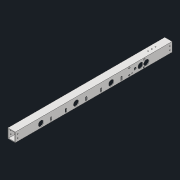
# Autodesk Inventor part: Left Frame
Saved by Autodesk Inventor 2022 (Build 260153000, 153)
## iProperties
Created: 2022-09-06
Part Number: Left Frame
Material: Generic
Document SubType Name: Modeling
Designer: robpl
Density: 1 g/cm^3
Appearance: Default
Author: robpl
Autodesk Inventor part; units mm, degrees
ref_plane "YZ Plane" through (0, 0, 0) normal (1, 0, 0) x (0, 1, 0)
ref_plane "XZ Plane" through (0, 0, 0) normal (0, 1, 0) x (-1, 0, 0)
sketch "Sketch1" plane through (0, 0, 0) normal (0, 0, 1) x (1, 0, 0)
  line L0 (0, 0) -> (40, 0)
  line L1 (40, 0) -> (40, 50)
  line L2 (40, 50) -> (0, 50)
  line L3 (0, 50) -> (0, 0)
  line L4 (37, 47) -> (37, 3)
  line L5 (37, 3) -> (3, 3)
  line L6 (3, 3) -> (3, 47)
  line L7 (3, 47) -> (37, 47)
  dimension "d0" = 40
  dimension "d1" = 50
  dimension "d2" = 3
  constraints: 16 end point, 4 parallel, 2 perpendicular, 1 horizontal, 3 other
  measures "d0" distance of L2.end L1.end
  measures "d1" distance of L1.end L0.end
  measures "d2" distance between parallel lines of L1 L4
extrude "Extrusion1" add sketch "Sketch1" along normal blind 850
sketch "Sketch2" plane through (40, 0, 0) normal (1, 0, 0) x (0, 0, -1)
  line L0 (0, 0) -> (0, 50) projected
  line L1 (0, 50) -> (-850, 50) projected
  line L2 (-850, 0) -> (-850, 50) projected
  line L3 (0, 0) -> (-850, 0) projected
  point P0 (-710.75, 21)
  point P1 (-520.25, 21)
  point P2 (-329.75, 21)
  point P3 (-139.25, 21)
  dimension "d5" = 190.5
  dimension "d6" = 190.5
  dimension "d7" = 190.5
  dimension "d8" = 850
  dimension "d9" = 139.25
  dimension "d10" = 21
  constraints: 3 horizontal alignment
  measures "d5" distance of point (-329.75, 21) point (-139.25, 21)
  measures "d6" distance of point (-520.25, 21) point (-329.75, 21)
  measures "d7" distance of point (-710.75, 21) point (-520.25, 21)
  measures "d8" distance of L0.end L1.end
  measures "d9" distance from line of point (-139.25, 21) L0
  measures "d10" distance from line of L3 point (-139.25, 21)
hole "Hole1" at (40, 21, 710.75) at (40, 21, 520.25) at (40, 21, 329.75) at (40, 21, 139.25) direction (-1, 0, 0) diameter 28.575 end through all
sketch "Sketch3" plane through (0, 0, 0) normal (0, -1, 0) x (1, 0, 0)
  line L0 (37, 0) -> (37, 850) projected
  line L1 (3, 0) -> (3, 850) projected
  line L2 (37, 755) -> (3, 755)
  line L3 (3, 755) -> (3, 95)
  line L4 (3, 95) -> (37, 95)
  line L5 (37, 95) -> (37, 755)
  line L6 (40, 725.0375) -> (40, 696.4625) projected
  line L7 (40, 0) -> (40, 850) projected
  line L8 (0, 850) -> (40, 850) projected
  line L9 (0, 0) -> (40, 0) projected
  point P0 (40, 710.75)
  point P1 (37, 95)
  point P2 (3, 755)
  dimension "d18" = 28.575
  dimension "d19" = 14.2875
  dimension "d22" = 95
  dimension "d23" = 95
  constraints: 8 end point, 3 point on line, 2 parallel, 1 horizontal, 1 perpendicular
  measures "d18" distance of L6.start L6.end
  measures "d19" distance of L6.start point (40, 710.75)
  measures "d22" distance between parallel lines of L8 L2
  measures "d23" distance between parallel lines of L9 L4
extrude "Extrusion2" cut sketch "Sketch3" against normal blind 3 contours L4 L1 L2 L0
sketch "Sketch4" plane through (40, 0, 0) normal (1, 0, 0) x (0, 0, -1)
  line L0 (-842.1969, 39.5285) -> (-10.8553, 39.5285)
  line L1 (-10.8553, 39.5285) -> (-10.8553, 6.7172)
  line L2 (-10.8553, 6.7172) -> (-842.1969, 6.7172)
  line L3 (-842.1969, 6.7172) -> (-842.1969, 39.5285)
  point P0 (0, 0)
  constraints: 8 end point, 2 parallel, 1 horizontal, 1 perpendicular
extrude "Extrusion3" [suppressed]
sketch "Sketch5" plane through (0, 0, 0) normal (-1, 0, 0) x (0, 0, 1)
  line L0 (0, 50) -> (0, 0) projected
  line L1 (0, 0) -> (850, 0) projected
  circle A0 centre (710.75, 21) radius 14.2875 projected
  circle A1 centre (139.25, 21) radius 14.2875 projected
  circle A2 centre (329.75, 21) radius 14.2875 projected
  circle A3 centre (520.25, 21) radius 14.2875 projected
  line L2 (0, 0) -> (0, 50) projected
  line L3 (0, 50) -> (850, 50) projected
  line L4 (850, 0) -> (850, 50) projected
  line L5 (0, 0) -> (850, 0) projected
  line L6 (139.25, 21) -> (107.5, 22.8)
  dimension "d37" = 31.801
  dimension "d39" = 107.5
  dimension "d41" = 22.8
  constraints: 2 end point, 1 coincident
  measures "d37" distance of L6.start L6.end
  measures "d39" distance from line of L0 L6.end
  measures "d41" distance from line of L1 L6.end
hole "Hole2" at (0, 22.8, 107.5) direction (1, 0, 0) diameter 28.575 end through all
sketch "Sketch6" plane through (40, 0, 0) normal (1, 0, 0) x (0, 0, -1)
  circle A0 centre (-107.5, 22.8) radius 14.2875 projected
  circle A1 centre (-329.75, 21) radius 14.2875 projected
  circle A2 centre (-710.75, 21) radius 14.2875 projected
  circle A3 centre (-520.25, 21) radius 14.2875 projected
  circle A4 centre (-139.25, 21) radius 14.2875 projected
  line L0 (0, 3) -> (0, 47) projected
  line L1 (0, 47) -> (-850, 47) projected
  line L2 (-850, 3) -> (-850, 47) projected
  line L3 (-755, 3) -> (-850, 3) projected
  line L4 (-755, 0) -> (-755, 3) projected
  line L5 (-95, 0) -> (-755, 0) projected
  line L6 (-95, 0) -> (-95, 3) projected
  line L7 (0, 3) -> (-95, 3) projected
  point P0 (0, 0)
  point P1 (-78.24, 22.8)
  dimension "d42" = 29.26
  constraints: 1 horizontal alignment
  measures "d42" distance of A0.centre point (-78.24, 22.8)
hole "Hole3" at (40, 22.8, 78.24) direction (-1, 0, 0) diameter 13 end through all
sketch "Sketch9" plane through (40, 0, 0) normal (1, 0, 0) x (0, 0, -1)
  point P0 (0, 0)
  point P1 (-127.5, 42)
  point P2 (-46.5, 42)
  point P3 (-46.5, 8)
  point P4 (-125.5, 5)
  dimension "d78" = 5
  dimension "d79" = 8
  dimension "d80" = 42
  dimension "d81" = 46.5
  dimension "d82" = 81
  dimension "d83" = 79
  constraints: 1 horizontal alignment, 1 vertical alignment
  measures "d78" vertical distance of point (0, 0) point (-125.5, 5)
  measures "d79" vertical distance of point (0, 0) point (-46.5, 8)
  measures "d80" vertical distance of point (0, 0) point (-46.5, 42)
  measures "d81" horizontal distance of point (0, 0) point (-46.5, 8)
  measures "d82" horizontal distance of point (-127.5, 42) point (-46.5, 8)
  measures "d83" horizontal distance of point (-125.5, 5) point (-46.5, 8)
hole "Hole7" at (40, 42, 127.5) at (40, 42, 46.5) at (40, 8, 46.5) at (40, 5, 125.5) direction (-1, 0, 0) diameter 9 depth 8 tip angle 118
sketch "Sketch10" plane through (3, 3, 0) normal (1, 0, 0) x (0, 0, -1)
  circle A0 centre (-125.5, 2) radius 4.5 projected
  circle A1 centre (-127.5, 39) radius 4.5 projected
  circle A2 centre (-46.5, 39) radius 4.5 projected
  circle A3 centre (-46.5, 5) radius 4.5 projected
  point P0 (0, -3)
  constraints: 4 coincident
hole "Hole8" at (3, 5, 125.5) at (3, 42, 127.5) at (3, 42, 46.5) at (3, 8, 46.5) direction (-1, 0, 0) diameter 4 end through all countersink diameter 9 countersink angle 90
sketch "Sketch11" plane through (0, 0, 0) normal (0, -1, 0) x (1, 0, 0)
  point P0 (0, 0)
  point P1 (20, 51.5)
  point P2 (20, 86.5)
  dimension "d98" = 35
  dimension "d99" = 51.5
  dimension "d100" = 20
  constraints: 1 vertical alignment
  measures "d98" distance of point (20, 51.5) point (20, 86.5)
  measures "d99" vertical distance of point (0, 0) point (20, 51.5)
  measures "d100" horizontal distance of point (0, 0) point (20, 51.5)
hole "Hole9" at (20, 0, 51.5) at (20, 0, 86.5) direction (0, 1, 0) diameter 6 depth 8 tip angle 118
sketch "Sketch12" plane through (40, 0, 0) normal (1, 0, 0) x (0, 0, -1)
  point P0 (0, 0)
  point P1 (-12.5, 15)
  point P2 (-12.5, 35)
  point P3 (-837.5, 35)
  point P4 (-837.5, 15)
  dimension "d108" = 12.5
  dimension "d109" = 35
  dimension "d110" = 15
  dimension "d111" = 837.5
  constraints: 2 horizontal alignment, 2 vertical alignment
  measures "d108" horizontal distance of point (-12.5, 35) point (0, 0)
  measures "d109" vertical distance of point (0, 0) point (-12.5, 35)
  measures "d110" vertical distance of point (0, 0) point (-12.5, 15)
  measures "d111" horizontal distance of point (0, 0) point (-837.5, 15)
hole "Hole10" at (40, 15, 12.5) at (40, 35, 12.5) at (40, 35, 837.5) at (40, 15, 837.5) direction (-1, 0, 0) diameter 6 end through all
sketch "Sketch13" plane through (0, 0, 0) normal (-1, 0, 0) x (0, 0, 1)
  line L0 (0, 0) -> (850, 0) projected
  point P0 (245, 12.5)
  point P1 (425, 12.5)
  point P2 (605, 12.5)
  dimension "d119" = 180
  dimension "d120" = 180
  dimension "d121" = 12.5
  dimension "d122" = 425
  constraints: 2 horizontal alignment
  measures "d119" distance of point (425, 12.5) point (605, 12.5)
  measures "d120" distance of point (245, 12.5) point (425, 12.5)
  measures "d121" distance from line of L0 point (245, 12.5)
  measures "d122" horizontal distance of L0.start point (425, 12.5)
hole "Hole11" at (0, 12.5, 245) at (0, 12.5, 425) at (0, 12.5, 605) direction (1, 0, 0) diameter 5 depth 8 tip angle 118
sketch "Sketch14" plane through (40, 0, 0) normal (1, 0, 0) x (0, 0, -1)
  line L0 (-655.75, 21) -> (-655.75, 8) construction
  line L1 (-659.75, 21) -> (-659.75, 8)
  line L2 (-651.75, 8) -> (-651.75, 21)
  arc A0 (-651.75, 21) -> (-659.75, 21) centre (-655.75, 21) ccw
  arc A1 (-659.75, 8) -> (-651.75, 8) centre (-655.75, 8) ccw
  line L3 (0, 0) -> (-850, 0) projected
  circle A2 centre (-837.5, 35) radius 3 projected
  circle A3 centre (-12.5, 15) radius 3 projected
  circle A4 centre (-12.5, 35) radius 3 projected
  circle A5 centre (-837.5, 15) radius 3 projected
  circle A6 centre (-46.5, 8) radius 4.5 projected
  circle A7 centre (-127.5, 42) radius 4.5 projected
  circle A8 centre (-46.5, 42) radius 4.5 projected
  circle A9 centre (-125.5, 5) radius 4.5 projected
  circle A10 centre (-78.24, 22.8) radius 6.5 projected
  circle A11 centre (-107.5, 22.8) radius 14.2875 projected
  circle A12 centre (-329.75, 21) radius 14.2875 projected
  circle A13 centre (-710.75, 21) radius 14.2875 projected
  circle A14 centre (-520.25, 21) radius 14.2875 projected
  circle A15 centre (-139.25, 21) radius 14.2875 projected
  line L4 (0, 0) -> (0, 50) projected
  line L5 (0, 50) -> (-850, 50) projected
  line L6 (-850, 0) -> (-850, 50) projected
  line L7 (0, 0) -> (-850, 0) projected
  line L8 (-575.25, 21) -> (-575.25, 8) construction
  line L9 (-571.25, 21) -> (-571.25, 8)
  line L10 (-579.25, 8) -> (-579.25, 21)
  arc A16 (-571.25, 21) -> (-579.25, 21) centre (-575.25, 21) ccw
  arc A17 (-579.25, 8) -> (-571.25, 8) centre (-575.25, 8) ccw
  line L11 (-465.25, 8) -> (-465.25, 21) construction
  line L12 (0, 47) -> (-850, 47) projected
  line L13 (-461.25, 8) -> (-461.25, 21)
  line L14 (-469.25, 21) -> (-469.25, 8)
  arc A18 (-469.25, 8) -> (-461.25, 8) centre (-465.25, 8) ccw
  arc A19 (-461.25, 21) -> (-469.25, 21) centre (-465.25, 21) ccw
  line L15 (-384.75, 8) -> (-384.75, 21) construction
  line L16 (-388.75, 8) -> (-388.75, 21)
  line L17 (-380.75, 21) -> (-380.75, 8)
  arc A20 (-388.75, 8) -> (-380.75, 8) centre (-384.75, 8) ccw
  arc A21 (-380.75, 21) -> (-388.75, 21) centre (-384.75, 21) ccw
  line L18 (-274.75, 21) -> (-274.75, 8) construction
  line L19 (-270.75, 21) -> (-270.75, 8)
  line L20 (-278.75, 8) -> (-278.75, 21)
  arc A22 (-270.75, 21) -> (-278.75, 21) centre (-274.75, 21) ccw
  arc A23 (-278.75, 8) -> (-270.75, 8) centre (-274.75, 8) ccw
  line L21 (-194.25, 21) -> (-194.25, 8) construction
  line L22 (-190.25, 21) -> (-190.25, 8)
  line L23 (-198.25, 8) -> (-198.25, 21)
  arc A24 (-190.25, 21) -> (-198.25, 21) centre (-194.25, 21) ccw
  arc A25 (-198.25, 8) -> (-190.25, 8) centre (-194.25, 8) ccw
  point P0 (-655.75, 14.5)
  point P1 (-575.25, 14.5)
  point P2 (-465.25, 14.5)
  point P3 (-384.75, 14.5)
  point P4 (-274.75, 14.5)
  point P5 (-194.25, 14.5)
  dimension "d130" = 8
  dimension "d131" = 8
  dimension "d132" = 21
  dimension "d133" = 55
  dimension "d134" = 55
  dimension "d135" = 55
  dimension "d136" = 55
  dimension "d137" = 55
  dimension "d138" = 55
  constraints: 48 end point, 24 point on circle, 24 tangent, 14 parallel, 12 centre point, 6 midpoint, 5 equal radius, 5 horizontal alignment, 2 vertical, 1 perpendicular
  measures "d130" diameter of A1
  measures "d131" distance from line of L3 L0.end
  measures "d132" distance from line of L3 L0.start
  measures "d133" distance from line of L0 A13.centre
  measures "d134" horizontal distance of A14.centre point (-575.25, 14.5)
  measures "d135" distance from line of L11 A14.centre
  measures "d136" horizontal distance of A12.centre L15.start
  measures "d137" horizontal distance of A12.centre point (-274.75, 14.5)
  measures "d138" horizontal distance of A15.centre point (-194.25, 14.5)
extrude "Extrusion4" cut sketch "Sketch14" against normal through all contours A0 L2 A1 L1 | L9 A17 L10 A16 | A18 L14 A19 L13 | L16 A21 L17 A20 | L19 A23 L20 A22
ref_plane "Work Plane1" through (0, 0, 139.25) normal (0, 0, -1) x (-1, 0, 0)
mirror "Two Motors" about plane through (0, 0, 139.25) normal (0, 0, -1) of "Hole2", "Hole3", "Hole7", "Hole8"
sketch "Sketch16" plane through (40, 0, 0) normal (1, 0, 0) x (0, 0, -1)
  point P0 (0, 0)
  point P1 (-216.5, 10)
  dimension "d144" = 216.5
  dimension "d145" = 10
  measures "d144" horizontal distance of point (0, 0) point (-216.5, 10)
  measures "d145" vertical distance of point (0, 0) point (-216.5, 10)
hole "Two Motors b" at (40, 10, 216.5) direction (-1, 0, 0) diameter 6 end through all
sketch "Sketch18" plane through (40, 0, 0) normal (1, 0, 0) x (0, 0, -1)
  circle A0 centre (-216.5, 10) radius 3 projected
  circle A1 centre (-153, 5) radius 4.5 projected
  circle A2 centre (-232, 42) radius 4.5 projected
  circle A3 centre (-151, 42) radius 4.5 projected
  circle A4 centre (-232, 8) radius 4.5 projected
  circle A5 centre (-171, 22.8) radius 14.2875 projected
  circle A6 centre (-200.26, 22.8) radius 6.5 projected
  line L0 (-469.25, 8) -> (-469.25, 21) projected
  arc A7 (-461.25, 21) -> (-469.25, 21) centre (-465.25, 21) ccw projected
  line L1 (-461.25, 21) -> (-461.25, 8) projected
  arc A8 (-469.25, 8) -> (-461.25, 8) centre (-465.25, 8) ccw projected
  arc A9 (-388.75, 8) -> (-380.75, 8) centre (-384.75, 8) ccw projected
  line L2 (-388.75, 8) -> (-388.75, 21) projected
  arc A10 (-380.75, 21) -> (-388.75, 21) centre (-384.75, 21) ccw projected
  line L3 (-380.75, 21) -> (-380.75, 8) projected
  arc A11 (-571.25, 21) -> (-579.25, 21) centre (-575.25, 21) ccw projected
  line L4 (-571.25, 21) -> (-571.25, 8) projected
  arc A12 (-579.25, 8) -> (-571.25, 8) centre (-575.25, 8) ccw projected
  line L5 (-579.25, 8) -> (-579.25, 21) projected
  arc A13 (-270.75, 21) -> (-278.75, 21) centre (-274.75, 21) ccw projected
  line L6 (-270.75, 21) -> (-270.75, 8) projected
  arc A14 (-278.75, 8) -> (-270.75, 8) centre (-274.75, 8) ccw projected
  line L7 (-278.75, 8) -> (-278.75, 21) projected
  line L8 (-651.75, 21) -> (-651.75, 8) projected
  arc A15 (-659.75, 8) -> (-651.75, 8) centre (-655.75, 8) ccw projected
  line L9 (-659.75, 8) -> (-659.75, 21) projected
  arc A16 (-651.75, 21) -> (-659.75, 21) centre (-655.75, 21) ccw projected
  circle A17 centre (-837.5, 35) radius 3 projected
  circle A18 centre (-12.5, 15) radius 3 projected
  circle A19 centre (-12.5, 35) radius 3 projected
  circle A20 centre (-837.5, 15) radius 3 projected
  circle A21 centre (-46.5, 8) radius 4.5 projected
  circle A22 centre (-127.5, 42) radius 4.5 projected
  circle A23 centre (-46.5, 42) radius 4.5 projected
  circle A24 centre (-125.5, 5) radius 4.5 projected
  circle A25 centre (-78.24, 22.8) radius 6.5 projected
  circle A26 centre (-107.5, 22.8) radius 14.2875 projected
  circle A27 centre (-329.75, 21) radius 14.2875 projected
  circle A28 centre (-710.75, 21) radius 14.2875 projected
  circle A29 centre (-520.25, 21) radius 14.2875 projected
  circle A30 centre (-139.25, 21) radius 14.2875 projected
  line L10 (0, 0) -> (0, 50) projected
  line L11 (0, 50) -> (-850, 50) projected
  line L12 (-850, 0) -> (-850, 50) projected
  line L13 (0, 0) -> (-850, 0) projected
extrude "Extrusion6" add sketch "Sketch18" against normal blind 3 contours A21 | A22 | A23 | A24 | A25 | A26
sketch "Sketch19" plane through (3, 3, 0) normal (1, 0, 0) x (0, 0, -1)
  circle A0 centre (-216.5, 7) radius 3 projected
  circle A1 centre (-153, 2) radius 4.5 projected
  circle A2 centre (-151, 39) radius 4.5 projected
  circle A3 centre (-232, 5) radius 4.5 projected
  circle A4 centre (-232, 39) radius 4.5 projected
  circle A5 centre (-171, 19.8) radius 14.2875 projected
  circle A6 centre (-200.26, 19.8) radius 6.5 projected
  line L0 (-469.25, 5) -> (-469.25, 18) projected
  arc A7 (-461.25, 18) -> (-469.25, 18) centre (-465.25, 18) ccw projected
  line L1 (-461.25, 18) -> (-461.25, 5) projected
  arc A8 (-469.25, 5) -> (-461.25, 5) centre (-465.25, 5) ccw projected
  arc A9 (-388.75, 5) -> (-380.75, 5) centre (-384.75, 5) ccw projected
  line L2 (-388.75, 5) -> (-388.75, 18) projected
  arc A10 (-380.75, 18) -> (-388.75, 18) centre (-384.75, 18) ccw projected
  line L3 (-380.75, 18) -> (-380.75, 5) projected
  arc A11 (-571.25, 18) -> (-579.25, 18) centre (-575.25, 18) ccw projected
  line L4 (-571.25, 18) -> (-571.25, 5) projected
  arc A12 (-579.25, 5) -> (-571.25, 5) centre (-575.25, 5) ccw projected
  line L5 (-579.25, 5) -> (-579.25, 18) projected
  arc A13 (-270.75, 18) -> (-278.75, 18) centre (-274.75, 18) ccw projected
  line L6 (-270.75, 18) -> (-270.75, 5) projected
  arc A14 (-278.75, 5) -> (-270.75, 5) centre (-274.75, 5) ccw projected
  line L7 (-278.75, 5) -> (-278.75, 18) projected
  line L8 (-651.75, 18) -> (-651.75, 5) projected
  arc A15 (-659.75, 5) -> (-651.75, 5) centre (-655.75, 5) ccw projected
  line L9 (-659.75, 5) -> (-659.75, 18) projected
  arc A16 (-651.75, 18) -> (-659.75, 18) centre (-655.75, 18) ccw projected
  circle A17 centre (-425, 9.5) radius 2.5 projected
  circle A18 centre (-245, 9.5) radius 2.5 projected
  circle A19 centre (-605, 9.5) radius 2.5 projected
  circle A20 centre (-837.5, 32) radius 3 projected
  circle A21 centre (-12.5, 12) radius 3 projected
  circle A22 centre (-12.5, 32) radius 3 projected
  circle A23 centre (-837.5, 12) radius 3 projected
  circle A24 centre (-46.5, 39) radius 4.5 projected
  circle A25 centre (-125.5, 2) radius 4.5 projected
  circle A26 centre (-127.5, 39) radius 4.5 projected
  circle A27 centre (-46.5, 5) radius 4.5 projected
  circle A28 centre (-78.24, 19.8) radius 6.5 projected
  circle A29 centre (-107.5, 19.8) radius 14.2875 projected
  circle A30 centre (-329.75, 18) radius 14.2875 projected
  circle A31 centre (-710.75, 18) radius 14.2875 projected
  circle A32 centre (-520.25, 18) radius 14.2875 projected
  circle A33 centre (-139.25, 18) radius 14.2875 projected
  line L10 (0, 0) -> (0, 44) projected
  line L11 (0, 44) -> (-850, 44) projected
  line L12 (-850, 0) -> (-850, 44) projected
  line L13 (-755, 0) -> (-850, 0) projected
  line L14 (-755, -3) -> (-755, 0) projected
  line L15 (-95, -3) -> (-755, -3) projected
  line L16 (-95, -3) -> (-95, 0) projected
  line L17 (0, 0) -> (-95, 0) projected
  point P0 (0, -3)
extrude "Extrusion7" add sketch "Sketch19" against normal blind 3 contours A24 | A25 | A26 | A27 | A28 | A29
sketch "Sketch20" plane through (0, 50, 0) normal (0, 1, 0) x (1, 0, 0)
  point P0 (0, 0)
  point P1 (20, -110)
  point P2 (20, -90)
  point P3 (20, -70)
  dimension "d168" = 70
  dimension "d169" = 20
  dimension "d170" = 20
  dimension "d171" = 20
  constraints: 2 vertical alignment
  measures "d168" vertical distance of point (0, 0) point (20, -70)
  measures "d169" distance of point (20, -90) point (20, -70)
  measures "d170" distance of point (20, -110) point (20, -90)
  measures "d171" horizontal distance of point (0, 0) point (20, -70)
hole "Hole14" at (20, 50, 110) at (20, 50, 90) at (20, 50, 70) direction (0, -1, 0) diameter 5 depth 8 tip angle 118
equation "\"d6\" = d5"
equation "\"d7\" = d5"
equation "\"d9\" = -1.5 * d5 + 0.5 * d8"
equation "\"d19\" = 0.5 * d18"
equation "\"d120\" = d119"
equation "\"d134\" = d133"
equation "\"d135\" = d133"
equation "\"d136\" = d133"
equation "\"d137\" = d133"
equation "\"d138\" = d133"
equation "\"d170\" = d169"
body "Solid1"
